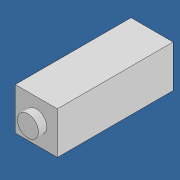
# Autodesk Inventor part: Diode_Laser
Saved by Autodesk Inventor 2020 (Build 240168000, 168)
## iProperties
Created: 2021-07-14
Part Number: Diode_Laser
Material: 一般
Document SubType Name: Modeling
Designer: ken113
Density: 1 g/cm^3
Appearance: 既定
Author: ken113
Autodesk Inventor part; units mm, degrees
ref_plane "YZ Plane" through (0, 0, 0) normal (1, 0, 0) x (0, 1, 0)
ref_plane "XZ Plane" through (0, 0, 0) normal (0, 1, 0) x (-1, 0, 0)
ref_plane "XY Plane" through (0, 0, 0) normal (0, 0, 1) x (1, 0, 0)
sketch "スケッチ1" plane through (0, 0, 0) normal (0, 0, 1) x (1, 0, 0)
  line L0 (-20, -20) -> (20, -20)
  line L1 (20, -20) -> (20, 20)
  line L2 (20, 20) -> (-20, 20)
  line L3 (-20, 20) -> (-20, -20)
  line L4 (-20, -20) -> (20, 20) construction
  line L5 (20, -20) -> (-20, 20) construction
  point P0 (0, 0)
  dimension "d0" = 40
  dimension "d1" = 40
  constraints: 12 end point, 2 midpoint, 2 parallel, 1 horizontal, 1 perpendicular
  measures "d0" distance of L2.end L1.end
  measures "d1" distance of L1.end L0.end
extrude "押し出し1" add sketch "スケッチ1" along normal blind 110
sketch "スケッチ2" plane through (0, 0, 110) normal (0, 0, 1) x (1, 0, 0)
  circle A0 centre (0, 0) radius 10
  dimension "d4" = 20
  constraints: 1 centre point, 1 coincident
  measures "d4" diameter of A0
extrude "押し出し2" add sketch "スケッチ2" along normal blind 8
sketch "スケッチ3" plane through (-20, -20, 0) normal (-1, 0, 0) x (0, 0, 1)
  line L0 (0, 40) -> (0, 0) projected
  line L1 (0, 0) -> (110, 0) projected
  line L2 (110, 40) -> (110, 0) projected
  line L3 (0, 40) -> (110, 40) projected
  line L4 (64, 10) -> (104, 10)
  line L5 (104, 10) -> (104, 30)
  line L6 (104, 30) -> (64, 30)
  line L7 (64, 30) -> (64, 10)
  line L8 (64, 10) -> (104, 30) construction
  line L9 (104, 10) -> (64, 30) construction
  point P0 (0, 20)
  point P1 (84, 20)
  point P2 (0, 20)
  point P3 (84, 20)
  dimension "d7" = 20
  dimension "d8" = 40
  dimension "d9" = 6
  constraints: 12 end point, 4 midpoint, 2 parallel, 1 horizontal, 1 horizontal alignment, 1 perpendicular
  measures "d7" distance of L4.end L5.end
  measures "d8" distance of L5.end L6.end
  measures "d9" distance between parallel lines of L2 L5
hole "穴1" at (-20, 10, 64) at (-20, -10, 64) at (-20, -10, 104) at (-20, 10, 104) direction (1, 0, 0) diameter 3.3 depth 8.8
